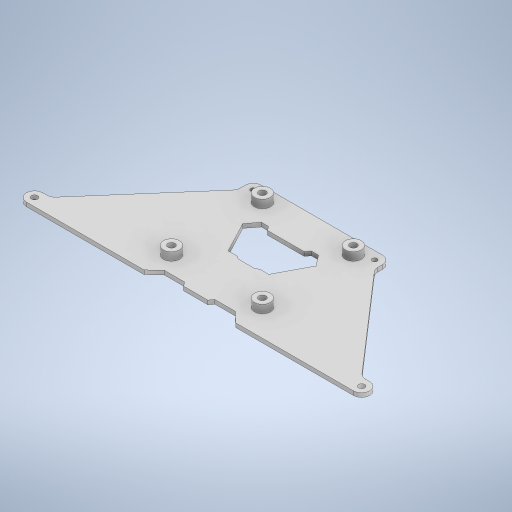
# Autodesk Inventor part: ElectronicsMount - BoltOnStyle
Saved by Autodesk Inventor 2023 (Build 270158000, 158)
## iProperties
Created: 2022-12-11
Part Number: ElectronicsMount - BoltOnStyle
Material: Generic
Document SubType Name: Modeling
Designer: Administrator
Density: 1 g/cm^3
Appearance: Default
Author: Administrator
Autodesk Inventor part; units mm, degrees
ref_plane "YZ Plane" through (0, 0, 0) normal (1, 0, 0) x (0, 1, 0)
ref_plane "XZ Plane" through (0, 0, 0) normal (0, 1, 0) x (-1, 0, 0)
ref_plane "XY Plane" through (0, 0, 0) normal (0, 0, 1) x (1, 0, 0)
sketch "Sketch1" plane through (0, 0, 0) normal (0, 1, 0) x (-1, 0, 0)
  circle A0 centre (-13, 3.6355) radius 1.25
  circle A1 centre (47, 3.6355) radius 1.25
  circle A2 centre (-63.9, 60.95) radius 1.55
  circle A3 centre (-63.9, 60.95) radius 1.5
  circle A4 centre (97.9, 60.95) radius 1.55
  circle A5 centre (97.9, 60.95) radius 1.5
  arc A6 (47, -0.3645) -> (51, 3.6355) centre (47, 3.6355) ccw
  arc A7 (-17, 3.6355) -> (-13, -0.3645) centre (-13, 3.6355) ccw
  arc A8 (-63.9, 64.95) -> (-63.9, 56.95) centre (-63.9, 60.95) ccw
  arc A9 (97.9, 56.95) -> (97.9, 64.95) centre (97.9, 60.95) ccw
  line L0 (-13, -0.3645) -> (47, -0.3645)
  line L1 (-63.9, 64.95) -> (97.9, 64.95)
  line L2 (-17, 3.6355) -> (-17, 6.1391)
  line L3 (51, 3.6355) -> (51, 6.1391)
  arc A10 (51, 3.6355) -> (47, -0.3645) centre (47, 3.6355) ccw construction
  arc A11 (-13, -0.3645) -> (-17, 3.6355) centre (-13, 3.6355) ccw construction
  line L4 (-63.9, 56.95) -> (-61.722, 56.95)
  line L5 (97.9, 56.95) -> (95.722, 56.95)
  line L6 (92.7041, 55.5753) -> (51.9821, 8.7645)
  line L7 (-58.7041, 55.5753) -> (-17.9821, 8.7645)
  arc A12 (-58.7041, 55.5753) -> (-61.722, 56.95) centre (-61.722, 52.95) ccw
  arc A13 (95.722, 56.95) -> (92.7041, 55.5753) centre (95.722, 52.95) ccw
  arc A14 (51.9821, 8.7645) -> (51, 6.1391) centre (55, 6.1391) ccw
  arc A15 (-17, 6.1391) -> (-17.9821, 8.7645) centre (-21, 6.1391) ccw
  arc A16 (-63.9, 56.95) -> (-63.9, 64.95) centre (-63.9, 60.95) ccw construction
  arc A17 (97.9, 64.95) -> (97.9, 56.95) centre (97.9, 60.95) ccw construction
  point P0 (0, 0)
  point P1 (17, 90.5)
  dimension "d0" = 2.5
  dimension "d1" = 2.5
  dimension "d2" = 3
  dimension "d3" = 3
  dimension "d4" = 8
  dimension "d5" = 8
  dimension "d6" = 8
  dimension "d7" = 8
  dimension "d8" = 60
  dimension "d18" = 4
  constraints: 24 point on circle, 18 centre point, 16 end point, 10 tangent, 5 coincident, 3 equal radius, 2 horizontal, 2 vertical
  measures "d0" diameter of A0
  measures "d1" diameter of A1
  measures "d2" diameter of A3
  measures "d3" diameter of A5
  measures "d4" diameter of A6
  measures "d5" diameter of A7
  measures "d6" diameter of A8
  measures "d7" diameter of A9
  measures "d8" distance of A1.centre A0.centre
  measures "d18" radius of A12
extrude "Extrusion1" add sketch "Sketch1" along normal blind 2 contours L0 A7 L2 A15 L7 A12 L4 A8 L1 A9 L5 A13 L6 A14 L3 A6
sketch "Sketch2" plane through (0, 2, 0) normal (0, 1, 0) x (1, 0, 0)
  circle A0 centre (13, -3.6355) radius 1.25 projected
  circle A1 centre (-47, -3.6355) radius 1.25 projected
  circle A2 centre (-39.5, -6.6355) radius 4
  circle A3 centre (5.5, -6.6355) radius 4
  circle A4 centre (5.5, -51.6355) radius 4
  circle A5 centre (-39.5, -51.6355) radius 4
  line L0 (13, 0.3645) -> (-47, 0.3645) projected
  circle A6 centre (-39.5, -6.6355) radius 1.75
  circle A7 centre (5.5, -6.6355) radius 1.75
  circle A8 centre (5.5, -51.6355) radius 1.75
  circle A9 centre (-39.5, -51.6355) radius 1.75
  point P0 (0, 0)
  dimension "d21" = 60
  dimension "d22" = 8
  dimension "d23" = 8
  dimension "d24" = 8
  dimension "d25" = 8
  dimension "d26" = 45
  dimension "d27" = 45
  dimension "d28" = 45
  dimension "d29" = 7
  dimension "d30" = 45
  dimension "d31" = 7.5
  dimension "d32" = 3.5
  dimension "d33" = 3.5
  dimension "d34" = 3.5
  dimension "d35" = 3.5
  constraints: 8 centre point, 4 coincident, 1 horizontal alignment, 1 vertical alignment
  measures "d21" distance of A0.centre A1.centre
  measures "d22" diameter of A2
  measures "d23" diameter of A3
  measures "d24" diameter of A4
  measures "d25" diameter of A5
  measures "d26" distance of A3.centre A2.centre
  measures "d27" distance of A2.centre A5.centre
  measures "d28" distance of A4.centre A5.centre
  measures "d29" distance from line of A3.centre L0
  measures "d30" distance of A4.centre A3.centre
  measures "d31" horizontal distance of A0.centre A3.centre
  measures "d32" diameter of A6
  measures "d33" diameter of A7
  measures "d34" diameter of A8
  measures "d35" diameter of A9
extrude "Extrusion2" add sketch "Sketch2" along normal blind 4 contours A2 | A3 | A4 | A5
sketch "Sketch3" plane through (0, 2, 0) normal (0, 1, 0) x (1, 0, 0)
  circle A0 centre (13, -3.6355) radius 1.55 construction
  line L0 (13, -3.6355) -> (-2, 2) construction
  line L1 (-2, 2) -> (-2, 4) construction
  line L2 (-2, 2) -> (-2, 4) construction
  line L3 (-2, 4) -> (6, 6.8723) construction
  line L4 (9.8, 6.8723) -> (53.9673, -18.6277) construction
  line L5 (6, 6.8723) -> (9.8, 6.8723) construction
  line L6 (9.8, 6.8723) -> (53.9673, -18.6277) construction
  line L7 (57.4673, -24.6899) -> (57.0036, -33.6779) construction
  line L8 (53.9673, -18.6277) -> (57.4673, -24.6899) construction
  line L9 (57.4673, -24.6899) -> (57.0036, -33.6779) construction
  line L10 (75.376, -65.5) -> (80.5, -65.5) construction
  line L11 (57.0036, -33.6779) -> (75.376, -65.5) construction
  line L12 (75.376, -65.5) -> (6.5, -65.7) construction
  line L13 (6.5, -65.7) -> (6.2893, -65.5) construction
  line L14 (0.6, -60.1) -> (-9.5, -60.1)
  line L15 (-9.5, -60.1) -> (-11, -62.1)
  line L16 (-9.5, -60.1) -> (-11, -62.1)
  line L17 (-23, -62.1) -> (-11, -62.1)
  line L18 (-11, -62.1) -> (-23, -62.1)
  line L19 (-24.5, -60.1) -> (-23, -62.1)
  line L20 (-23, -62.1) -> (-24.5, -60.1)
  line L21 (-34.6, -60.1) -> (-24.5, -60.1)
  line L22 (-24.5, -60.1) -> (-34.6, -60.1)
  line L23 (-40.5, -71.9) -> (-40.5, -65.7) construction
  line L24 (-34.6, -60.1) -> (-39.7098, -64.95)
  line L25 (-114.5, -65.5) -> (-109.376, -65.5) construction
  line L26 (-40.5, -65.7) -> (-109.376, -65.5) construction
  line L27 (-109.376, -65.5) -> (-91.0036, -33.6779) construction
  line L28 (-87.9673, -18.6277) -> (-91.4673, -24.6899) construction
  line L29 (-91.0036, -33.6779) -> (-91.4673, -24.6899) construction
  line L30 (-91.4673, -24.6899) -> (-87.9673, -18.6277) construction
  line L31 (-40, 6.8723) -> (-43.8, 6.8723) construction
  line L32 (-87.9673, -18.6277) -> (-43.8, 6.8723) construction
  line L33 (-43.8, 6.8723) -> (-40, 6.8723) construction
  line L34 (-32, 4) -> (-40, 6.8723) construction
  line L35 (-40, 6.8723) -> (-32, 4) construction
  line L36 (-32, 4) -> (-32, 2) construction
  line L37 (-32, 2) -> (-2, 2) construction
  line L38 (-6.4, -15.5) -> (-2.8831, -15.5)
  line L39 (-2.8831, -15.5) -> (-6.4, -15.5)
  line L40 (-26.1, -17.5) -> (-7.9, -17.5)
  line L41 (-6.4, -15.5) -> (-7.9, -17.5)
  line L42 (-7.9, -17.5) -> (-26.1, -17.5)
  line L43 (-31.1169, -15.5) -> (-27.6, -15.5)
  line L44 (-26.1, -17.5) -> (-27.6, -15.5)
  line L45 (-35.1306, -20.7029) -> (-31.1169, -15.5)
  line L46 (-27.6, -15.5) -> (-31.1169, -15.5)
  line L47 (-31.1169, -15.5) -> (-35.1306, -20.7029)
  line L48 (-35.1306, -20.7029) -> (-27.0449, -36)
  line L49 (-22.7189, -36) -> (-27.0449, -36)
  line L50 (-27.0449, -36) -> (-22.7189, -36)
  line L51 (-20.9689, -37) -> (-22.7189, -36)
  line L52 (-22.7189, -36) -> (-20.9689, -37)
  line L53 (-13.0311, -37) -> (-20.9689, -37)
  line L54 (-20.9689, -37) -> (-13.0311, -37)
  line L55 (-11.2811, -36) -> (-13.0311, -37)
  line L56 (-13.0311, -37) -> (-11.2811, -36)
  line L57 (-6.9551, -36) -> (-11.2811, -36)
  line L58 (-11.2811, -36) -> (-6.9551, -36)
  line L59 (1.1306, -20.7029) -> (-6.9551, -36)
  line L60 (-6.9551, -36) -> (1.1306, -20.7029)
  line L61 (1.1306, -20.7029) -> (-2.8831, -15.5)
  circle A1 centre (13, -3.6355) radius 1.25 projected
  line L62 (-97.9, -64.95) -> (63.9, -64.95) projected
  line L63 (5.7098, -64.95) -> (-39.7098, -64.95)
  line L64 (5.7098, -64.95) -> (0.6, -60.1)
  point P0 (0, 0)
  point P1 (17, 90.5)
  constraints: 128 end point, 15 collinear, 5 perpendicular, 4 parallel, 3 point on line, 1 centre point, 1 coincident
extrude "Extrusion3" cut sketch "Sketch3" against normal up to next contours L64 L62 L24 L21 L19 L17 L15 L14 | L38 L61 L59 L57 L55 L53 L51 L49 L48 L45 L43 L44 L40 L41
equation "\"d31\" = -0.5 * d26 + 0.5 * d21"
body "Solid1"
